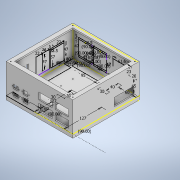
# Autodesk Inventor part: bakeoutbox
Saved by Autodesk Inventor 2020.2 (Build 242310000, 310)
## iProperties
Created: 2020-01-31
Part Number: bakeoutbox
Material: Generic
Document SubType Name: Modeling
Designer: ColinP
Density: 1 g/cm^3
Appearance: Default
Author: ColinP
Autodesk Inventor part; units mm, degrees
ref_plane "YZ Plane" through (0, 0, 0) normal (1, 0, 0) x (0, 1, 0)
ref_plane "XZ Plane" through (0, 0, 0) normal (0, 1, 0) x (-1, 0, 0)
ref_plane "XY Plane" through (0, 0, 0) normal (0, 0, 1) x (1, 0, 0)
sketch "Sketch14" plane through (0, 0, 0) normal (0, 1, 0) x (-1, 0, 0)
  line L0 (225, 225) -> (0, 225)
  line L1 (0, 225) -> (0, 0)
  line L2 (0, 0) -> (225, 0)
  line L3 (225, 0) -> (225, 225)
  dimension "d298" = 225
  dimension "d299" = 225
  constraints: 8 end point, 2 parallel, 1 horizontal, 1 perpendicular
  measures "d298" distance of L1.end L2.end
  measures "d299" distance of L0.end L1.end
extrude "Extrusion8" add sketch "Sketch14" along normal blind 12.7
sketch "Sketch15" plane through (0, 12.7, 0) normal (0, 1, 0) x (1, 0, 0)
  line L0 (0, 0) -> (-225, 0) projected
  line L1 (-225, 0) -> (-225, -225) projected
  line L2 (-225, -225) -> (0, -225) projected
  line L3 (0, -225) -> (0, 0) projected
  line L4 (0, -225) -> (0, 0) projected
  line L5 (0, -225) -> (0, -221)
  line L6 (0, -221) -> (-4, -221)
  line L7 (-4, -221) -> (-4, -4)
  line L8 (-4, -4) -> (-221, -4)
  line L9 (0, 0) -> (-225, 0) projected
  line L10 (-221, -4) -> (-221, -221)
  line L11 (-221, -221) -> (-4, -221)
  dimension "d130" = 4
  dimension "d131" = 4
  dimension "d132" = 217
  dimension "d133" = 217
  dimension "d134" = 90
  constraints: 12 end point, 2 perpendicular, 2 point on line, 1 parallel
  measures "d130" distance of L2.end L5.end
  measures "d131" distance of L5.end L6.end
  measures "d132" distance of L6.end L7.end
  measures "d133" distance of L7.end L8.end
  measures "d134" angle of L8 L7
extrude "Extrusion9" add sketch "Sketch15" along normal blind 100
sketch "Sketch16" plane through (-225, 0, 225) normal (0, 0, 1) x (1, 0, 0)
  line L0 (4, 12.7) -> (110.4, 12.7)
  line L1 (221, 12.7) -> (4, 12.7) projected
  line L2 (110.4, 12.7) -> (110.4, 22.7)
  line L3 (110.4, 22.7) -> (155.7, 22.7)
  line L4 (155.7, 22.7) -> (155.7, 45.4)
  line L5 (155.7, 45.4) -> (110.4, 45.4)
  line L6 (110.4, 45.4) -> (110.4, 22.7)
  line L7 (155.7, 22.7) -> (165.7, 22.7)
  line L8 (165.7, 22.7) -> (165.7, 45.4)
  line L9 (165.7, 45.4) -> (211, 45.4)
  line L10 (211, 45.4) -> (211, 22.7)
  line L11 (211, 22.7) -> (165.7, 22.7)
  line L12 (211, 45.4) -> (211, 55.4)
  line L13 (211, 55.4) -> (211, 78.1)
  line L14 (211, 78.1) -> (165.7, 78.1)
  line L15 (165.7, 78.1) -> (165.7, 55.4)
  line L16 (165.7, 55.4) -> (211, 55.4)
  line L17 (155.7, 45.4) -> (155.7, 55.4)
  line L18 (155.7, 78.1) -> (155.7, 55.4)
  line L19 (110.4, 55.4) -> (155.7, 55.4)
  line L20 (110.4, 55.4) -> (110.4, 78.1)
  line L21 (155.7, 78.1) -> (110.4, 78.1)
  point P0 (225, 0)
  dimension "d138" = 106.4
  dimension "d139" = 10
  dimension "d140" = 45.3
  dimension "d141" = 22.7
  dimension "d142" = 10
  dimension "d143" = 45.3
  dimension "d144" = 10
  dimension "d145" = 22.7
  constraints: 42 end point, 17 point on line, 10 perpendicular, 2 collinear, 1 horizontal
  measures "d138" distance of L0.start L0.end
  measures "d139" distance of L0.end L2.end
  measures "d140" distance of L2.end L3.end
  measures "d141" distance of L3.end L4.end
  measures "d142" distance of L3.end L7.end
  measures "d143" distance of L8.end L9.end
  measures "d144" distance of L9.end L12.end
  measures "d145" distance of L12.end L13.end
extrude "Extrusion10" cut sketch "Sketch16" against normal blind 10
sketch "Sketch17" plane through (-225, 0, 225) normal (0, 0, 1) x (1, 0, 0)
  line L0 (221, 12.7) -> (221, 112.7) projected
  line L1 (221, 12.7) -> (73.4, 12.7)
  line L2 (4, 12.7) -> (221, 12.7) projected
  line L3 (73.4, 12.7) -> (73.4, 22.7)
  line L4 (73.4, 22.7) -> (56.7, 22.7)
  line L5 (56.7, 22.7) -> (56.7, 35.6)
  line L6 (56.7, 35.6) -> (73.4, 35.6)
  line L7 (73.4, 35.6) -> (73.4, 22.7)
  line L8 (56.7, 35.6) -> (56.7, 45.6)
  line L9 (56.7, 45.6) -> (73.4, 45.6)
  line L10 (73.4, 45.6) -> (73.4, 58.5)
  line L11 (73.4, 58.5) -> (56.7, 58.5)
  line L12 (56.7, 58.5) -> (56.7, 45.6)
  line L13 (56.7, 45.6) -> (40.7, 45.6)
  line L14 (40.7, 45.6) -> (40.7, 58.5)
  line L15 (40.7, 58.5) -> (24, 58.5)
  line L16 (24, 58.5) -> (24, 45.6)
  line L17 (24, 45.6) -> (40.7, 45.6)
  line L18 (40.7, 35.6) -> (40.7, 22.7)
  line L19 (24, 22.7) -> (40.7, 22.7)
  line L20 (24, 22.7) -> (24, 35.6)
  line L21 (40.7, 35.6) -> (24, 35.6)
  point P0 (225, 0)
  dimension "d148" = 147.6
  dimension "d149" = 10
  dimension "d150" = 16.7
  dimension "d151" = 12.9
  dimension "d152" = 10
  dimension "d153" = 12.9
  dimension "d154" = 16
  dimension "d155" = 16.7
  constraints: 40 end point, 17 point on line, 12 perpendicular, 1 horizontal
  measures "d148" distance of L0.start L1.end
  measures "d149" distance of L1.end L3.end
  measures "d150" distance of L3.end L4.end
  measures "d151" distance of L4.end L5.end
  measures "d152" distance of L5.end L8.end
  measures "d153" distance of L9.end L10.end
  measures "d154" distance of L8.end L13.end
  measures "d155" distance of L14.end L15.end
sketch "Sketch18" plane through (-225, 0, 225) normal (0, 0, 1) x (1, 0, 0)
  line L0 (24, 58.5) -> (24, 45.6) projected
  line L1 (40.7, 45.6) -> (40.7, 58.5) projected
  line L2 (56.7, 58.5) -> (56.7, 45.6) projected
  line L3 (73.4, 45.6) -> (73.4, 58.5) projected
  line L4 (73.4, 35.6) -> (73.4, 22.7) projected
  line L5 (56.7, 22.7) -> (56.7, 35.6) projected
  line L6 (40.7, 35.6) -> (40.7, 22.7) projected
  line L7 (24, 22.7) -> (24, 35.6) projected
  line L8 (24, 52.05) -> (21, 52.05)
  line L9 (24, 29.15) -> (21, 29.15)
  line L10 (40.7, 29.15) -> (43.7, 29.15)
  line L11 (40.7, 52.05) -> (43.7, 52.05)
  line L12 (56.7, 52.05) -> (53.7, 52.05)
  line L13 (56.7, 29.15) -> (53.7, 29.15)
  line L14 (73.4, 52.05) -> (76.4, 52.05)
  line L15 (76.4, 52.05) -> (76.4, 29.15)
  point P0 (225, 0)
  dimension "d156" = 3
  dimension "d157" = 3
  dimension "d158" = 3
  dimension "d159" = 3
  dimension "d160" = 3
  constraints: 16 end point, 7 horizontal, 7 midpoint, 1 perpendicular
  measures "d156" distance of L8.start L8.end
  measures "d157" distance of L10.start L10.end
  measures "d158" distance of L11.start L11.end
  measures "d159" distance of L12.start L12.end
  measures "d160" distance of L14.start L14.end
hole "Hole5" at (-204, 52.05, 225) at (-204, 29.15, 225) at (-181.3, 29.15, 225) at (-181.3, 52.05, 225) at (-171.3, 52.05, 225) at (-171.3, 29.15, 225) at (-148.6, 29.15, 225) at (-148.6, 52.05, 225) direction (0, 0, -1) diameter 3 depth 8.865
extrude "Extrusion11" cut sketch "Sketch17" against normal blind 10
sketch "Sketch19" plane through (-225, 0, 0) normal (-1, 0, 0) x (0, 0, 1)
  line L0 (221, 12.7) -> (4, 12.7) projected
  line L1 (4, 12.7) -> (154, 12.7)
  line L2 (154, 12.7) -> (154, 22.7)
  line L3 (154, 22.7) -> (166.5, 22.7)
  line L4 (166.5, 22.7) -> (166.5, 45.2)
  line L5 (166.5, 45.2) -> (154, 45.2)
  line L6 (154, 45.2) -> (154, 22.7)
  line L7 (166.5, 45.2) -> (171.5, 45.2)
  line L8 (171.5, 45.2) -> (171.5, 22.7)
  line L9 (171.5, 22.7) -> (184, 22.7)
  line L10 (184, 22.7) -> (184, 45.2)
  line L11 (184, 45.2) -> (171.5, 45.2)
  line L12 (184, 45.2) -> (189, 45.2)
  line L13 (189, 45.2) -> (189, 22.7)
  line L14 (189, 22.7) -> (201.5, 22.7)
  line L15 (201.5, 22.7) -> (201.5, 45.2)
  line L16 (201.5, 45.2) -> (189, 45.2)
  point P0 (0, 0)
  dimension "d170" = 150
  dimension "d171" = 10
  dimension "d172" = 12.5
  dimension "d173" = 22.5
  dimension "d174" = 5
  dimension "d175" = 12.5
  dimension "d176" = 5
  dimension "d177" = 12.5
  constraints: 32 end point, 10 perpendicular, 9 point on line, 1 horizontal
  measures "d170" distance of L0.end L1.end
  measures "d171" distance of L1.end L2.end
  measures "d172" distance of L2.end L3.end
  measures "d173" distance of L3.end L4.end
  measures "d174" distance of L4.end L7.end
  measures "d175" distance of L8.end L9.end
  measures "d176" distance of L10.end L12.end
  measures "d177" distance of L13.end L14.end
extrude "Extrusion12" cut sketch "Sketch19" against normal blind 10
sketch "Sketch20" plane through (-225, 0, 0) normal (-1, 0, 0) x (0, 0, 1)
  line L0 (154, 45.2) -> (166.5, 45.2) projected
  line L1 (154, 45.2) -> (4, 45.2)
  line L2 (4, 12.7) -> (4, 112.7) projected
  line L3 (4, 45.2) -> (4, 55.2)
  line L4 (4, 55.2) -> (154, 55.2)
  line L5 (154, 55.2) -> (154, 72)
  line L6 (154, 72) -> (162.2, 72)
  line L7 (162.2, 72) -> (162.2, 55.2)
  line L8 (162.2, 55.2) -> (154, 55.2)
  line L9 (162.2, 55.2) -> (168.4, 55.2)
  line L10 (168.4, 55.2) -> (168.4, 72)
  line L11 (168.4, 72) -> (176.6, 72)
  line L12 (176.6, 72) -> (176.6, 55.2)
  line L13 (176.6, 55.2) -> (168.4, 55.2)
  line L14 (176.6, 55.2) -> (182.8, 55.2)
  line L15 (182.8, 55.2) -> (182.8, 72)
  line L16 (182.8, 72) -> (191, 72)
  line L17 (191, 72) -> (191, 55.2)
  line L18 (191, 55.2) -> (182.8, 55.2)
  line L19 (191, 55.2) -> (197.2, 55.2)
  line L20 (197.2, 55.2) -> (197.2, 72)
  line L21 (197.2, 72) -> (205.4, 72)
  line L22 (205.4, 72) -> (205.4, 55.2)
  line L23 (205.4, 55.2) -> (197.2, 55.2)
  point P0 (0, 0)
  dimension "d180" = 10
  dimension "d181" = 150
  dimension "d182" = 16.8
  dimension "d183" = 8.2
  dimension "d184" = 6.2
  dimension "d185" = 8.2
  dimension "d186" = 6.2
  dimension "d187" = 8.2
  dimension "d188" = 6.2
  dimension "d189" = 8.2
  constraints: 44 end point, 14 point on line, 13 perpendicular, 1 horizontal, 1 vertical
  measures "d180" distance of L1.end L3.end
  measures "d181" distance of L3.end L4.end
  measures "d182" distance of L4.end L5.end
  measures "d183" distance of L5.end L6.end
  measures "d184" distance of L7.end L9.end
  measures "d185" distance of L10.end L11.end
  measures "d186" distance of L12.end L14.end
  measures "d187" distance of L15.end L16.end
  measures "d188" distance of L17.end L19.end
  measures "d189" distance of L20.end L21.end
extrude "Extrusion13" cut sketch "Sketch20" against normal blind 10
sketch "Sketch24" plane through (0, 0, 0) normal (0, 0, -1) x (-1, 0, 0)
  line L0 (4, 12.7) -> (221, 12.7) projected
  line L1 (4, 12.7) -> (104, 12.7)
  line L2 (104, 12.7) -> (129, 12.7)
  line L3 (129, 12.7) -> (129, 32.7)
  line L4 (129, 32.7) -> (156.5, 32.7)
  line L5 (156.5, 32.7) -> (179, 32.7)
  line L6 (179, 32.7) -> (179, 79.7)
  line L7 (129, 32.7) -> (129, 79.7)
  point P0 (0, 0)
  dimension "d226" = 100
  dimension "d227" = 25
  dimension "d228" = 20
  dimension "d229" = 27.5
  dimension "d230" = 90
  dimension "d231" = 22.5
  dimension "d232" = 47
  dimension "d233" = 47
  constraints: 14 end point, 2 perpendicular, 2 point on line, 2 vertical, 1 horizontal
  measures "d226" distance of L0.start L1.end
  measures "d227" distance of L1.end L2.end
  measures "d228" distance of L2.end L3.end
  measures "d229" distance of L3.end L4.end
  measures "d230" angle of L3 L4
  measures "d231" distance of L4.end L5.end
  measures "d232" distance of L5.end L6.end
  measures "d233" distance of L3.end L7.end
hole "Hole8" at (-129, 79.7, 0) at (-129, 32.7, 0) at (-179, 32.7, 0) at (-179, 79.7, 0) direction (0, 0, 1) diameter 3.302 depth 12.3 thread size "8-32 UNC" class "2B" standard "ANSI Unified Screw Threads"
sketch "Sketch26" plane through (-221, 12.7, 4) normal (0, 0, 1) x (1, 0, 0)
  circle A0 centre (42, 67) radius 1.651 projected
  line L0 (42, 67) -> (64.5, 67)
  line L1 (64.5, 67) -> (69.5, 67)
  circle A1 centre (92, 67) radius 1.651 projected
  line L2 (69.5, 67) -> (92, 67)
  line L3 (92, 67) -> (114.5, 67)
  line L4 (114.5, 67) -> (114.5, 20)
  line L5 (114.5, 20) -> (69.5, 20)
  line L6 (69.5, 20) -> (64.5, 20)
  line L7 (64.5, 20) -> (19.5, 20)
  line L8 (19.5, 20) -> (19.5, 67)
  line L9 (19.5, 67) -> (42, 67)
  line L10 (-4, 100) -> (221, 100) projected
  line L11 (64.5, 67) -> (64.5, 20)
  line L12 (69.5, 67) -> (69.5, 20)
  line L13 (69.5, 67) -> (116.5, 67) construction
  line L14 (19.5, 67) -> (19.5, 72)
  line L15 (19.5, 72) -> (64.5, 72)
  line L16 (64.5, 72) -> (64.5, 15)
  line L17 (64.5, 15) -> (19.5, 15)
  line L18 (19.5, 15) -> (19.5, 20)
  line L19 (69.5, 67) -> (69.5, 72)
  line L20 (69.5, 72) -> (114.5, 72)
  line L21 (114.5, 72) -> (114.5, 15)
  line L22 (114.5, 15) -> (69.5, 15)
  line L23 (69.5, 20) -> (69.5, 15)
  point P0 (221, -12.7)
  dimension "d249" = 22.5
  dimension "d250" = 5
  dimension "d251" = 22.5
  dimension "d252" = 47
  dimension "d253" = 90
  dimension "d254" = 45
  dimension "d255" = 90
  dimension "d256" = 5
  dimension "d257" = 180
  dimension "d258" = 45
  dimension "d259" = 180
  dimension "d260" = 47
  dimension "d261" = 90
  dimension "d262" = 47
  dimension "d263" = 47
  dimension "d264" = 90
  dimension "d273" = 5
  dimension "d274" = 57
  dimension "d275" = 90
  dimension "d276" = 5
  dimension "d277" = 57
  constraints: 46 end point, 8 perpendicular, 8 point on line, 3 collinear, 2 horizontal, 1 vertical
  measures "d249" distance of L0.start L0.end
  measures "d250" distance of L0.end L1.end
  measures "d251" distance of L2.end L3.end
  measures "d252" distance of L3.end L4.end
  measures "d253" angle of L3 L4
  measures "d254" distance of L4.end L5.end
  measures "d255" angle of L4 L5
  measures "d256" distance of L5.end L6.end
  measures "d257" angle of L6 L5
  measures "d258" distance of L6.end L7.end
  measures "d259" angle of L7 L6
  measures "d260" distance of L7.end L8.end
  measures "d261" angle of L7 L8
  measures "d262" distance of L0.end L6.end
  measures "d263" distance of L1.end L5.end
  measures "d264" angle of L12 L13
  measures "d273" distance of L8.end L14.end
  measures "d274" distance of L15.end L16.end
  measures "d275" angle of L15 L16
  measures "d276" distance of L1.end L19.end
  measures "d277" distance of L20.end L21.end
sketch "Sketch27" plane through (0, 12.7, 0) normal (0, 1, 0) x (1, 0, 0)
  line L0 (-114.6, -225) -> (-114.6, -98)
  line L1 (-114.6, -225) -> (12.4, -225) construction
  line L2 (-14, -225) -> (-14, -98)
  line L3 (-14, -225) -> (113, -225) construction
  line L4 (-14, -98) -> (-114.6, -98)
  point P0 (0, 0)
  dimension "d265" = 127
  dimension "d266" = 90
  dimension "d267" = 127
  dimension "d268" = 90
  constraints: 10 end point, 2 horizontal, 2 perpendicular, 2 vertical
  measures "d265" distance of L0.start L0.end
  measures "d266" angle of L1 L0
  measures "d267" distance of L2.start L2.end
  measures "d268" angle of L3 L2
sketch "Sketch32" plane through (0, 0, 225) normal (1, 0, 0) x (0, 0, -1)
  line L0 (221, 12.7) -> (221, 112.7) projected
  line L1 (221, 12.7) -> (221, 22.7)
  line L2 (221, 22.7) -> (206, 22.7)
  line L3 (206, 22.7) -> (140, 22.7)
  line L4 (140, 22.7) -> (140, 49.7)
  line L5 (140, 49.7) -> (206, 49.7)
  line L6 (206, 49.7) -> (206, 22.7)
  point P0 (225, 0)
  dimension "d308" = 10
  dimension "d309" = 15
  dimension "d310" = 66
  dimension "d311" = 27
  constraints: 12 end point, 2 parallel, 2 perpendicular, 1 horizontal, 1 point on line
  measures "d308" distance of L0.start L1.end
  measures "d309" distance of L1.end L2.end
  measures "d310" distance of L4.end L5.end
  measures "d311" distance of L3.end L4.end
sketch "Sketch33" plane through (-221, 5.2, 0) normal (-1, 0, 0) x (0, 0, 1)
  line L0 (4, 7.5) -> (4, 107.5) projected
  line L1 (4, 7.5) -> (34, 7.5)
  line L2 (221, 7.5) -> (4, 7.5) projected
  line L3 (34, 7.5) -> (34, 22.5)
  line L4 (34, 7.5) -> (49, 7.5) construction
  line L5 (34, 22.5) -> (34, 69.5)
  line L6 (34, 69.5) -> (56.5, 69.5)
  line L7 (56.5, 69.5) -> (79, 69.5)
  line L8 (79, 69.5) -> (79, 74.5)
  line L9 (79, 74.5) -> (34, 74.5)
  line L10 (34, 74.5) -> (34, 69.5)
  line L11 (79, 74.5) -> (79, 17.5)
  line L12 (79, 17.5) -> (34, 17.5)
  line L13 (56.5, 17.5) -> (56.5, 22.5)
  line L14 (79, 74.5) -> (84, 74.5)
  line L15 (84, 74.5) -> (106.5, 74.5)
  line L16 (106.5, 74.5) -> (129, 74.5)
  line L17 (129, 74.5) -> (129, 17.5)
  line L18 (129, 17.5) -> (84, 17.5)
  line L19 (84, 17.5) -> (84, 74.5)
  line L20 (106.5, 74.5) -> (106.5, 69.5)
  line L21 (106.5, 69.5) -> (106.5, 22.5)
  point P0 (0, -5.2)
  dimension "d312" = 30
  dimension "d313" = 15
  dimension "d314" = 90
  dimension "d327" = 47
  dimension "d328" = 22.5
  dimension "d329" = 22.5
  dimension "d330" = 5
  dimension "d331" = 57
  dimension "d332" = 5
  dimension "d333" = 5
  dimension "d334" = 22.5
  dimension "d335" = 22.5
  dimension "d336" = 5
  dimension "d337" = 47
  constraints: 40 end point, 8 perpendicular, 7 point on line, 5 vertical, 2 horizontal, 1 midpoint
  measures "d312" distance of L0.start L1.end
  measures "d313" distance of L1.end L3.end
  measures "d314" angle of L4 L3
  measures "d327" distance of L3.end L5.end
  measures "d328" distance of L5.end L6.end
  measures "d329" distance of L6.end L7.end
  measures "d330" distance of L7.end L8.end
  measures "d331" distance of L8.end L11.end
  measures "d332" distance of L13.start L13.end
  measures "d333" distance of L8.end L14.end
  measures "d334" distance of L14.end L15.end
  measures "d335" distance of L15.end L16.end
  measures "d336" distance of L15.end L20.end
  measures "d337" distance of L20.end L21.end
hole "Hole9" at (-221, 74.7, 56.5) at (-221, 27.7, 56.5) at (-221, 27.7, 106.5) at (-221, 74.7, 106.5) direction (-1, 0, 0) diameter 3.302 depth 12.3 thread size "8-32 UNC" class "2B" standard "ANSI Unified Screw Threads"
sketch "Sketch29" plane through (0, 12.7, 0) normal (0, 1, 0) x (1, 0, 0)
  line L0 (-201.5, -4) -> (-201.5, -26.86)
  line L1 (-4, -4) -> (-221, -4) projected
  line L2 (-201.5, -4) -> (-178.64, -4) construction
  line L3 (-201.5, -26.86) -> (-106.5, -26.86)
  line L4 (-106.5, -26.86) -> (-106.5, -4)
  line L5 (-221, -34) -> (-198, -34)
  line L6 (-198, -34) -> (-198, -129)
  line L7 (-198, -129) -> (-221, -129)
  point P0 (0, 0)
  point P1 (-106.5, -4)
  dimension "d286" = 22.86
  dimension "d287" = 90
  dimension "d288" = 95
  dimension "d289" = 90
  dimension "d346" = 23
  constraints: 14 end point, 5 perpendicular, 2 horizontal
  measures "d286" distance of L0.start L0.end
  measures "d287" angle of L0 L2
  measures "d288" distance of L0.end L3.end
  measures "d289" angle of L3 L0
  measures "d346" distance of L5.start L5.end
sketch "Sketch34" plane through (-221, 12.7, 4) normal (0, 0, 1) x (1, 0, 0)
  line L0 (217, 0) -> (0, 0) projected
  line L1 (217, 0) -> (217, 45)
  line L2 (217, 45) -> (197, 45)
  line L3 (197, 45) -> (197, 68)
  line L4 (197, 68) -> (135.4, 68)
  line L5 (135.4, 68) -> (135.4, 45)
  point P0 (221, -12.7)
  dimension "d347" = 45
  dimension "d348" = 20
  dimension "d349" = 23
  dimension "d350" = 61.6
  constraints: 10 end point, 4 perpendicular, 1 point on line, 1 vertical
  measures "d347" distance of L0.start L1.end
  measures "d348" distance of L1.end L2.end
  measures "d349" distance of L2.end L3.end
  measures "d350" distance of L3.end L4.end
hole "Hole10" at (-85.6, 80.7, 4) at (-24, 57.7, 4) direction (0, 0, -1) diameter 2.1565 depth 8.865 thread size "4-40 UNC" class "2B" standard "ANSI Unified Screw Threads"
extrude "Extrusion15" cut sketch "Sketch32" against normal blind 10
sketch "Sketch35" plane through (0, 0, 0) normal (0, 1, 0) x (1, 0, 0)
  line L0 (-221, -4) -> (-221, -221) projected
  line L1 (-221, -4) -> (-161, -4)
  line L2 (-4, -4) -> (-221, -4) projected
  line L3 (-161, -4) -> (-161, -64)
  line L4 (-161, -64) -> (-161, -104)
  line L5 (-4, -4) -> (-104, -4)
  line L6 (-104, -4) -> (-104, -64)
  line L7 (-104, -64) -> (-64, -64)
  line L8 (-4, -221) -> (-221, -221) projected
  line L9 (-221, -221) -> (-161, -221)
  line L10 (-161, -221) -> (-161, -141)
  line L11 (-161, -141) -> (-161, -181)
  point P0 (0, 0)
  dimension "d360" = 60
  dimension "d361" = 60
  dimension "d362" = 90
  dimension "d363" = 40
  dimension "d364" = 100
  dimension "d365" = 60
  dimension "d366" = 40
  dimension "d367" = 60
  dimension "d368" = 80
  dimension "d369" = 40
  constraints: 18 end point, 4 perpendicular, 4 point on line, 1 midpoint
  measures "d360" distance of L0.start L1.end
  measures "d361" distance of L1.end L3.end
  measures "d362" angle of L1 L3
  measures "d363" distance of L3.end L4.end
  measures "d364" distance of L2.start L5.end
  measures "d365" distance of L5.end L6.end
  measures "d366" distance of L6.end L7.end
  measures "d367" distance of L0.end L9.end
  measures "d368" distance of L9.end L10.end
  measures "d369" distance of L10.end L11.end
hole "Hole11" at (-161, 0, 141) at (-161, 0, 181) at (-161, 0, 104) at (-161, 0, 64) at (-104, 0, 64) at (-64, 0, 64) direction (0, 1, 0) diameter 3.429 end through all counterbore diameter 6 counterbore depth 4
sketch "Sketch36" plane through (-221, 12.7, 4) normal (0, 0, 1) x (1, 0, 0)
  line L0 (0, 100) -> (0, 95)
  line L1 (0, 95) -> (217, 95)
  line L2 (217, 95) -> (217, 100)
  line L3 (217, 100) -> (0, 100)
  point P0 (221, -12.7)
  dimension "d377" = 5
  dimension "d378" = 90
  constraints: 8 end point, 1 perpendicular, 1 vertical
  measures "d377" distance of L0.start L0.end
  measures "d378" angle of L1 L0
extrude "Extrusion16" add sketch "Sketch36" along normal blind 10
sketch "Sketch37" plane through (-221, 12.7, 221) normal (1, 0, 0) x (0, 0, -1)
  line L0 (0, 100) -> (0, 95)
  line L1 (217, 95) -> (207, 95) projected
  line L2 (0, 95) -> (207, 95)
  line L3 (207, 95) -> (207, 100) projected
  line L4 (207, 95) -> (207, 100)
  line L5 (207, 100) -> (0, 100)
  point P0 (221, -12.7)
  dimension "d381" = 5
  constraints: 8 end point, 1 perpendicular, 1 vertical
  measures "d381" distance of L0.start L0.end
extrude "Extrusion17" add sketch "Sketch37" along normal blind 10
sketch "Sketch38" plane through (-4, 12.7, 221) normal (0, 0, -1) x (-1, 0, 0)
  line L0 (0, 100) -> (0, 95)
  line L1 (207, 95) -> (207, 100) projected
  line L2 (0, 95) -> (207, 95)
  line L3 (207, 95) -> (207, 100)
  line L4 (207, 100) -> (0, 100)
  point P0 (-4, -12.7)
  dimension "d384" = 5
  constraints: 8 end point, 1 perpendicular, 1 vertical
  measures "d384" distance of L0.start L0.end
extrude "Extrusion18" add sketch "Sketch38" along normal blind 10
sketch "Sketch39" plane through (-4, 12.7, 4) normal (-1, 0, 0) x (0, 0, 1)
  line L0 (10, 100) -> (10, 95)
  line L1 (207, 95) -> (207, 100) projected
  line L2 (10, 95) -> (207, 95)
  line L3 (207, 95) -> (207, 100)
  line L4 (207, 100) -> (10, 100)
  point P0 (-4, -12.7)
  constraints: 8 end point, 3 perpendicular, 1 vertical
extrude "Extrusion19" add sketch "Sketch39" along normal blind 10
sketch "Sketch40" plane through (0, 112.7, 0) normal (0, 1, 0) x (1, 0, 0)
  line L0 (-225, 0) -> (-225, -225) projected
  line L1 (-225, -225) -> (-225, -217.5)
  line L2 (-225, -217.5) -> (-217.5, -217.5)
  line L3 (-217.5, -217.5) -> (-217.5, -7.5)
  line L4 (-217.5, -7.5) -> (-7.5, -7.5)
  line L5 (-7.5, -7.5) -> (-7.5, -217.5)
  line L6 (-4, -221) -> (-4, -4) projected
  line L7 (-7.5, -217.5) -> (-217.5, -217.5)
  point P0 (0, 0)
  dimension "d389" = 7.5
  dimension "d390" = 7.5
  dimension "d391" = 210
  dimension "d392" = 90
  dimension "d393" = 210
  dimension "d394" = 90
  dimension "d395" = 210
  dimension "d396" = 90
  constraints: 12 end point, 3 perpendicular, 1 parallel, 1 point on line
  measures "d389" distance of L0.end L1.end
  measures "d390" distance of L1.end L2.end
  measures "d391" distance of L2.end L3.end
  measures "d392" angle of L3 L2
  measures "d393" distance of L3.end L4.end
  measures "d394" angle of L3 L4
  measures "d395" distance of L4.end L5.end
  measures "d396" angle of L4 L5
hole "Hole12" at (-7.5, 112.7, 7.5) at (-217.5, 112.7, 7.5) at (-217.5, 112.7, 217.5) at (-7.5, 112.7, 217.5) direction (0, -1, 0) diameter 3.302 depth 12.3 thread size "8-32 UNC" class "2B" standard "ANSI Unified Screw Threads"
sketch "Sketch41" plane through (0, 12.7, 0) normal (0, 1, 0) x (1, 0, 0)
  line L0 (0, -225) -> (0, 0) projected
  line L1 (0, 0) -> (-60, 0)
  line L2 (0, 0) -> (-225, 0) projected
  line L3 (-60, 0) -> (-60, -40)
  line L4 (-60, -40) -> (-90, -40)
  line L5 (-225, -225) -> (-130, -225)
  line L6 (-225, -225) -> (0, -225) projected
  line L7 (-130, -225) -> (-130, -165)
  line L8 (-130, -165) -> (-130, -135)
  line L9 (-130, -135) -> (-130, -105)
  dimension "d404" = 60
  dimension "d405" = 40
  dimension "d406" = 30
  dimension "d414" = 95
  dimension "d415" = 60
  dimension "d416" = 30
  dimension "d417" = 30
  constraints: 14 end point, 3 perpendicular, 3 point on line, 1 vertical
  measures "d404" distance of L0.end L1.end
  measures "d405" distance of L1.end L3.end
  measures "d406" distance of L3.end L4.end
  measures "d414" distance of L5.start L5.end
  measures "d415" distance of L5.end L7.end
  measures "d416" distance of L7.end L8.end
  measures "d417" distance of L8.end L9.end
hole "Hole13" at (-60, 12.7, 40) at (-90, 12.7, 40) at (-130, 12.7, 165) at (-130, 12.7, 135) at (-130, 12.7, 105) direction (0, -1, 0) diameter 5.75 depth 10.979
body "Solid2"
